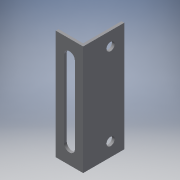
# Autodesk Inventor part: palmrest_L_large
Saved by Autodesk Inventor 2018 (Build 220112000, 112)
## iProperties
Created: 2018-04-05
Part Number: palmrest_L_large
Material: アルミニウム 6061
Document SubType Name: Modeling
Designer: NaMACHAN
Density: 2.7 g/cm^3
Appearance: アルミニウム - フラット
Author: NaMACHAN
Autodesk Inventor part; units mm, degrees
ref_plane "YZ Plane" through (0, 0, 0) normal (1, 0, 0) x (0, 1, 0)
ref_plane "XZ Plane" through (0, 0, 0) normal (0, 1, 0) x (-1, 0, 0)
ref_plane "XY Plane" through (0, 0, 0) normal (0, 0, 1) x (1, 0, 0)
sketch "スケッチ1" plane through (0, 0, 0) normal (1, 0, 0) x (0, 1, 0)
  line L0 (-5, -20) -> (5, -20)
  line L1 (5, -20) -> (5, 20)
  line L2 (5, 20) -> (-5, 20)
  line L3 (-5, 20) -> (-5, -20)
  line L4 (-5, -20) -> (5, 20) construction
  line L5 (5, -20) -> (-5, 20) construction
  point P0 (0, 0)
  dimension "d0" = 10
  dimension "d1" = 40
  constraints: 12 end point, 2 midpoint, 2 parallel, 1 horizontal, 1 perpendicular
  measures "d0" distance of L2.end L1.end
  measures "d1" distance of L1.end L0.end
extrude "押し出し1" add sketch "スケッチ1" along normal blind 10
shell "シェル1" thickness 1 removed faces 4 at (3.3333, 1.6667, 20) at (3.3333, 5, -6.6667) at (3.3333, -1.6667, -20) at (0, -1.6667, 6.6667)
sketch "スケッチ2" plane through (10, 0, 0) normal (1, 0, 0) x (0, 0, -1)
  line L0 (20, -5) -> (20, 5) projected
  line L1 (-20, 5) -> (-20, -5) projected
  line L2 (20, 5) -> (-20, 5) projected
  point P0 (0, 0)
  point P1 (-15, 0)
  point P2 (15, 0)
  dimension "d5" = 5
  dimension "d6" = 5
  dimension "d14" = 5
  constraints: 1 horizontal alignment
  measures "d5" distance from line of L0 point (15, 0)
  measures "d6" distance from line of L1 point (-15, 0)
  measures "d14" distance from line of L2 point (-15, 0)
hole "穴1" at (10, 0, 15) at (10, 0, -15) direction (-1, 0, 0) diameter 3 end through all
sketch "スケッチ3" plane through (0, -5, -20) normal (0, -1, 0) x (1, 0, 0)
  line L0 (7, 34) -> (7, 6)
  arc A0 (3, 6) -> (7, 6) centre (5, 6) ccw
  line L1 (3, 6) -> (3, 34)
  arc A1 (7, 34) -> (3, 34) centre (5, 34) ccw
  line L2 (0, 40) -> (10, 40) projected
  line L3 (0, 40) -> (0, 0) projected
  line L4 (0, 0) -> (10, 0) projected
  point P0 (0, 20)
  point P1 (3, 20)
  point P2 (0, 20)
  dimension "d15" = 2
  dimension "d17" = 5
  dimension "d22" = 6
  constraints: 4 end point, 4 point on circle, 4 tangent, 2 centre point, 2 midpoint, 2 vertical, 1 horizontal alignment
  measures "d15" radius of A1
  measures "d17" distance from line of L3 A1.centre
  measures "d22" distance from line of L2 A1.centre
extrude "押し出し2" cut sketch "スケッチ3" against normal blind 1
